Autodesk Fusion 360 part; units mm, degrees
(part 3 of 4)
  spline S239 degree 3 poles (-20.1278, 30.3585) (-20.2422, 30.4762) (-20.3885, 30.5351) (-20.5667, 30.5351) knots 0 0 0 0 1 1 1 1
  line L137 (-20.7879, 29.7232) -> (-20.24, 29.7232)
  spline S240 degree 3 poles (-20.24, 29.7232) (-20.2642, 29.6418) (-20.3043, 29.5768) (-20.3605, 29.5284) knots 0 0 0 0 1 1 1 1
  spline S241 degree 3 poles (-20.3605, 29.5284) (-20.4166, 29.48) (-20.4798, 29.4558) (-20.5502, 29.4558) knots 0 0 0 0 1 1 1 1
  spline S242 degree 3 poles (-20.5502, 29.4558) (-20.6493, 29.4558) (-20.7191, 29.485) (-20.7598, 29.5433) knots 0 0 0 0 1 1 1 1
  spline S243 degree 3 poles (-20.7598, 29.5433) (-20.8005, 29.6016) (-20.8099, 29.6616) (-20.7879, 29.7232) knots 0 0 0 0 1 1 1 1
  line L138 (-22.382, 30.5351) -> (-22.821, 30.4526)
  line L139 (-22.821, 30.4526) -> (-22.821, 30.3833)
  spline S244 degree 3 poles (-22.821, 30.3833) (-22.711, 30.3833) (-22.64, 30.3602) (-22.6081, 30.314) knots 0 0 0 0 1 1 1 1
  spline S245 degree 3 poles (-22.6081, 30.314) (-22.5762, 30.2678) (-22.5603, 30.1621) (-22.5603, 29.9971) knots 0 0 0 0 1 1 1 1
  line L140 (-22.5603, 29.9971) -> (-22.5603, 28.4426)
  line L141 (-22.5603, 28.4426) -> (-22.0652, 28.5251)
  line L142 (-22.0652, 28.5251) -> (-22.0652, 28.5944)
  spline S246 degree 3 poles (-22.0652, 28.5944) (-22.1752, 28.5944) (-22.2462, 28.6175) (-22.2781, 28.6637) knots 0 0 0 0 1 1 1 1
  spline S247 degree 3 poles (-22.2781, 28.6637) (-22.31, 28.7099) (-22.3259, 28.8155) (-22.3259, 28.9806) knots 0 0 0 0 1 1 1 1
  line L143 (-22.3259, 28.9806) -> (-22.3259, 29.5185)
  spline S248 degree 3 poles (-22.3259, 29.5185) (-22.2203, 29.3887) (-22.0861, 29.3238) (-21.9233, 29.3238) knots 0 0 0 0 1 1 1 1
  spline S249 degree 3 poles (-21.9233, 29.3238) (-21.767, 29.3238) (-21.6323, 29.3827) (-21.5189, 29.5004) knots 0 0 0 0 1 1 1 1
  spline S250 degree 3 poles (-21.5189, 29.5004) (-21.4056, 29.6181) (-21.349, 29.7606) (-21.349, 29.9278) knots 0 0 0 0 1 1 1 1
  spline S251 degree 3 poles (-21.349, 29.9278) (-21.349, 30.095) (-21.4056, 30.238) (-21.5189, 30.3569) knots 0 0 0 0 1 1 1 1
  spline S252 degree 3 poles (-21.5189, 30.3569) (-21.6323, 30.4757) (-21.767, 30.5351) (-21.9233, 30.5351) knots 0 0 0 0 1 1 1 1
  spline S253 degree 3 poles (-21.9233, 30.5351) (-22.0861, 30.5351) (-22.2214, 30.468) (-22.3292, 30.3338) knots 0 0 0 0 1 1 1 1
  spline S254 degree 3 poles (-22.3292, 30.3338) (-22.349, 30.435) (-22.3666, 30.5021) (-22.382, 30.5351) knots 0 0 0 0 1 1 1 1
  spline S255 degree 3 poles (-21.9926, 30.4031) (-21.8693, 30.4031) (-21.7758, 30.3591) (-21.712, 30.2711) knots 0 0 0 0 1 1 1 1
  spline S256 degree 3 poles (-21.712, 30.2711) (-21.6482, 30.183) (-21.6163, 30.0686) (-21.6163, 29.9278) knots 0 0 0 0 1 1 1 1
  spline S257 degree 3 poles (-21.6163, 29.9278) (-21.6163, 29.7892) (-21.6482, 29.6759) (-21.712, 29.5878) knots 0 0 0 0 1 1 1 1
  spline S258 degree 3 poles (-21.712, 29.5878) (-21.7758, 29.4998) (-21.8693, 29.4558) (-21.9926, 29.4558) knots 0 0 0 0 1 1 1 1
  spline S259 degree 3 poles (-21.9926, 29.4558) (-22.0652, 29.4558) (-22.1312, 29.4795) (-22.1906, 29.5268) knots 0 0 0 0 1 1 1 1
  spline S260 degree 3 poles (-22.1906, 29.5268) (-22.25, 29.5741) (-22.2951, 29.6374) (-22.3259, 29.7166) knots 0 0 0 0 1 1 1 1
  line L144 (-22.3259, 29.7166) -> (-22.3259, 30.1423)
  spline S261 degree 3 poles (-22.3259, 30.1423) (-22.2951, 30.2215) (-22.25, 30.2848) (-22.1906, 30.3321) knots 0 0 0 0 1 1 1 1
  spline S262 degree 3 poles (-22.1906, 30.3321) (-22.1312, 30.3794) (-22.0652, 30.4031) (-21.9926, 30.4031) knots 0 0 0 0 1 1 1 1
  line L145 (-23.9927, 30.5351) -> (-24.1379, 30.314)
  spline S263 degree 3 poles (-24.1379, 30.314) (-24.2413, 30.4614) (-24.3821, 30.5351) (-24.5604, 30.5351) knots 0 0 0 0 1 1 1 1
  spline S264 degree 3 poles (-24.5604, 30.5351) (-24.7166, 30.5351) (-24.8508, 30.4757) (-24.963, 30.3569) knots 0 0 0 0 1 1 1 1
  spline S265 degree 3 poles (-24.963, 30.3569) (-25.0752, 30.238) (-25.1314, 30.095) (-25.1314, 29.9278) knots 0 0 0 0 1 1 1 1
  spline S266 degree 3 poles (-25.1314, 29.9278) (-25.1314, 29.7606) (-25.0752, 29.6181) (-24.963, 29.5004) knots 0 0 0 0 1 1 1 1
  spline S267 degree 3 poles (-24.963, 29.5004) (-24.8508, 29.3827) (-24.7166, 29.3238) (-24.5604, 29.3238) knots 0 0 0 0 1 1 1 1
  spline S268 degree 3 poles (-24.5604, 29.3238) (-24.3975, 29.3238) (-24.2633, 29.3887) (-24.1577, 29.5185) knots 0 0 0 0 1 1 1 1
  line L146 (-24.1577, 29.5185) -> (-24.1577, 28.4426)
  line L147 (-24.1577, 28.4426) -> (-23.6626, 28.5251)
  line L148 (-23.6626, 28.5251) -> (-23.6626, 28.5944)
  spline S269 degree 3 poles (-23.6626, 28.5944) (-23.7726, 28.5944) (-23.8436, 28.6175) (-23.8755, 28.6637) knots 0 0 0 0 1 1 1 1
  spline S270 degree 3 poles (-23.8755, 28.6637) (-23.9074, 28.7099) (-23.9234, 28.8155) (-23.9234, 28.9806) knots 0 0 0 0 1 1 1 1
  line L149 (-23.9234, 28.9806) -> (-23.9234, 30.5351)
  line L150 (-23.9234, 30.5351) -> (-23.9927, 30.5351)
  spline S271 degree 3 poles (-24.4911, 30.4031) (-24.4162, 30.4031) (-24.3497, 30.3794) (-24.2914, 30.3321) knots 0 0 0 0 1 1 1 1
  spline S272 degree 3 poles (-24.2914, 30.3321) (-24.2331, 30.2848) (-24.1885, 30.2204) (-24.1577, 30.139) knots 0 0 0 0 1 1 1 1
  line L151 (-24.1577, 30.139) -> (-24.1577, 29.7166)
  spline S273 degree 3 poles (-24.1577, 29.7166) (-24.1885, 29.6374) (-24.2331, 29.5741) (-24.2914, 29.5268) knots 0 0 0 0 1 1 1 1
  spline S274 degree 3 poles (-24.2914, 29.5268) (-24.3497, 29.4795) (-24.4162, 29.4558) (-24.4911, 29.4558) knots 0 0 0 0 1 1 1 1
  spline S275 degree 3 poles (-24.4911, 29.4558) (-24.6143, 29.4558) (-24.7078, 29.4998) (-24.7716, 29.5878) knots 0 0 0 0 1 1 1 1
  spline S276 degree 3 poles (-24.7716, 29.5878) (-24.8354, 29.6759) (-24.8673, 29.7892) (-24.8673, 29.9278) knots 0 0 0 0 1 1 1 1
  spline S277 degree 3 poles (-24.8673, 29.9278) (-24.8673, 30.0686) (-24.8354, 30.183) (-24.7716, 30.2711) knots 0 0 0 0 1 1 1 1
  spline S278 degree 3 poles (-24.7716, 30.2711) (-24.7078, 30.3591) (-24.6143, 30.4031) (-24.4911, 30.4031) knots 0 0 0 0 1 1 1 1
  spline S279 degree 3 poles (-25.5637, 31.3701) (-25.6121, 31.3701) (-25.6528, 31.3294) (-25.6858, 31.248) knots 0 0 0 0 1 1 1 1
  line L152 (-25.6858, 31.248) -> (-26.3294, 29.6407)
  spline S280 degree 3 poles (-26.3294, 29.6407) (-26.3822, 29.5108) (-26.4604, 29.4459) (-26.5638, 29.4459) knots 0 0 0 0 1 1 1 1
  line L153 (-26.5638, 29.4459) -> (-26.5638, 29.3799)
  line L154 (-26.5638, 29.3799) -> (-26.1017, 29.3799)
  line L155 (-26.1017, 29.3799) -> (-26.1017, 29.4459)
  spline S281 degree 3 poles (-26.1017, 29.4459) (-26.1699, 29.4459) (-26.2106, 29.4597) (-26.2238, 29.4872) knots 0 0 0 0 1 1 1 1
  spline S282 degree 3 poles (-26.2238, 29.4872) (-26.237, 29.5147) (-26.2282, 29.5658) (-26.1974, 29.6407) knots 0 0 0 0 1 1 1 1
  line L156 (-26.1974, 29.6407) -> (-25.9862, 30.1687)
  line L157 (-25.9862, 30.1687) -> (-25.7452, 29.6407)
  spline S283 degree 3 poles (-25.7452, 29.6407) (-25.71, 29.5592) (-25.7001, 29.5064) (-25.7155, 29.4822) knots 0 0 0 0 1 1 1 1
  spline S284 degree 3 poles (-25.7155, 29.4822) (-25.7309, 29.458) (-25.7761, 29.4459) (-25.8509, 29.4459) knots 0 0 0 0 1 1 1 1
  line L158 (-25.8509, 29.4459) -> (-25.8509, 29.3799)
  line L159 (-25.8509, 29.3799) -> (-25.2667, 29.3799)
  line L160 (-25.2667, 29.3799) -> (-25.2667, 29.4459)
  spline S285 degree 3 poles (-25.2667, 29.4459) (-25.3173, 29.4459) (-25.358, 29.4597) (-25.3888, 29.4872) knots 0 0 0 0 1 1 1 1
  spline S286 degree 3 poles (-25.3888, 29.4872) (-25.4196, 29.5147) (-25.4526, 29.5658) (-25.4878, 29.6407) knots 0 0 0 0 1 1 1 1
  line L161 (-25.4878, 29.6407) -> (-25.8674, 30.4625)
  line L162 (-25.8674, 30.4625) -> (-25.7023, 30.875)
  spline S287 degree 3 poles (-25.7023, 30.875) (-25.6737, 30.9477) (-25.638, 31.0076) (-25.5951, 31.0549) knots 0 0 0 0 1 1 1 1
  spline S288 degree 3 poles (-25.5951, 31.0549) (-25.5522, 31.1022) (-25.5175, 31.1396) (-25.4911, 31.1671) knots 0 0 0 0 1 1 1 1
  spline S289 degree 3 poles (-25.4911, 31.1671) (-25.4647, 31.1946) (-25.4515, 31.226) (-25.4515, 31.2612) knots 0 0 0 0 1 1 1 1
  spline S290 degree 3 poles (-25.4515, 31.2612) (-25.4515, 31.2986) (-25.4631, 31.3261) (-25.4862, 31.3437) knots 0 0 0 0 1 1 1 1
  spline S291 degree 3 poles (-25.4862, 31.3437) (-25.5093, 31.3613) (-25.5351, 31.3701) (-25.5637, 31.3701) knots 0 0 0 0 1 1 1 1
  line L163 (-22, -1.425) -> (-22, 24.075)
  line L164 (-22, 24.075) -> (27.5, 24.075)
  line L165 (27.5, 24.075) -> (27.5, -1.425)
  line L166 (27.5, -1.425) -> (-22, -1.425)
  line L167 (53, -8.5) -> (53, 40.5)
  line L168 (53, 40.5) -> (-53, 40.5)
  line L169 (-53, 40.5) -> (-53, -8.5)
extrude "Extrude7" cut sketch "Sketch10" against normal blind 1 contours L1 L2 L3 S0 S1 L4 L5 L6 S2 S3 L7 L8 L9 L10 L11 S4 S5 S6 S7 | L12 S8 S9 S10 S11 S12 S13 L13 S14 S15 | L16 L17 L18 S19 S20 S21 S22 L19 L20 | L22 L23 L24 S27 S28 S29 S30 L25 L26 | S35 S36 S37 S38 S39 | L27 L28 L29 L30 L31 L32 L33 L34 L35 L36 L37 L38 L39 | L45 S51 S52 S54 S55 L48 | L40 S44 S45 L41 S46 S47 L42 L43 L44 L45 S54 S55 L48 | L42 S48 S49 S50 L43 L45 S51 S52 S53 L46 L47 L48 S56 S57 L49 S58 S59 | L42 S48 S49 S50 L43 L48 | S60 S61 L50 L51 S62 S63 S64 S65 S66 L52 L53 L54 S67 S68 S69 L55 L56 | S70 S71 L57 L58 S72 S73 S74 S75 S76 S77 L59 L60 S78 S79 S80 L61 L62 | S81 S82 L63 L64 S83 S84 S85 L65 L66 S86 S87 S88 L67 L68 | S89 S90 S91 L69 S92 S93 S94 S95 S96 L70 L71 S97 S98 S99 L72 | S100 S101 L73 L74 S102 S103 S104 L75 L76 S105 S106 S107 S108 L77 | S109 S110 S111 L78 S112 S113 S114 S115 S116 L79 L80 S117 S118 S119 L81 | S120 S121 L82 L83 S122 S123 S124 S125 S126 L84 L85 L86 S127 S128 S129 L87 L88 | S130 S131 S132 L89 S133 S134 S135 S136 S137 L90 L91 L92 S138 S139 S140 S141 L93 L94 | S142 S143 S144 L95 S145 S146 S147 L96 L97 S148 S149 S150 S151 L98 L99 bodies 8 in component "GNSS_Enclosure_Top"
hole "Hole4" at (-47.5, 30, 0) at (47.5, 30, 0) at (-47.5, -30, 0) at (47.5, -30, 0) direction (0, 0, -1) diameter 2.1 depth 4 tip angle 180 bodies 7 in component "GNSS_Enclosure_Bottom"
sketch "Sketch8 (2)" plane through (0, 0, 15.7) normal (0, 0, 1) x (-1, 0, 0) in component "GNSS_Enclosure_Bottom"
  line L0 (51, 30) -> (51, -30)
  arc A0 (47.5, -33.5) -> (51, -30) centre (47.5, -30) ccw
  arc A1 (47.5, -33.5) -> (46, -35) centre (47.5, -35) ccw
  arc A2 (42.5, -38.5) -> (46, -35) centre (42.5, -35) ccw
  line L1 (42.5, -38.5) -> (-42.5, -38.5)
  arc A3 (-46, -35) -> (-42.5, -38.5) centre (-42.5, -35) ccw
  arc A4 (-46, -35) -> (-47.5, -33.5) centre (-47.5, -35) ccw
  arc A5 (-51, -30) -> (-47.5, -33.5) centre (-47.5, -30) ccw
  line L2 (-51, -30) -> (-51, 30)
  arc A6 (-47.5, 33.5) -> (-51, 30) centre (-47.5, 30) ccw
  arc A7 (-47.5, 33.5) -> (-46, 35) centre (-47.5, 35) ccw
  arc A8 (-42.5, 38.5) -> (-46, 35) centre (-42.5, 35) ccw
  line L3 (-42.5, 38.5) -> (42.5, 38.5)
  arc A9 (46, 35) -> (42.5, 38.5) centre (42.5, 35) ccw
  arc A10 (46, 35) -> (47.5, 33.5) centre (47.5, 35) ccw
  arc A11 (51, 30) -> (47.5, 33.5) centre (47.5, 30) ccw
  line L4 (-53, -40.5) -> (53, -40.5)
  line L5 (53, -40.5) -> (53, 40.5)
  line L6 (53, 40.5) -> (-53, 40.5)
  line L7 (-53, 40.5) -> (-53, -40.5)
  line L8 (49.5, 37) -> (-49.5, 37)
  line L9 (-49.5, 37) -> (-49.5, -37)
  line L10 (-49.5, -37) -> (49.5, -37)
  line L11 (49.5, -37) -> (49.5, 37)
  point P0 (49.5, -37)
  point P1 (-49.5, -37)
  point P2 (-49.5, 37)
  point P3 (49.5, 37)
  constraint coincident P0 L10.end
  constraint coincident P1 L9.end
  constraint coincident P2 L8.end
  constraint coincident P3 L8.start
hole "Hole5" at (-49.5, 37, 15.7) at (-49.5, -37, 15.7) at (49.5, -37, 15.7) at (49.5, 37, 15.7) direction (0, 0, -1) diameter 2.1 depth 10 tip angle 180 bodies 7 in component "GNSS_Enclosure_Bottom"
fillet "Fillet1'" radius 2 8 edges at (53, -40.5, 5.35) (53, 0, -5) (0, -40.5, -5) (53, 40.5, 5.35) (0, 40.5, -5) (-53, 40.5, 5.35) (-53, 0, -5) (-53, -40.5, 5.35) on bodies 7 in component "GNSS_Enclosure_Bottom"
sketch "Sketch11" plane through (0, 0, 17.7) normal (0, 0, 1) x (-1, 0, 0) in component "GNSS_Enclosure_Top"
  spline S0 degree 3 poles (-34.0203, 31.3378) (-34.6769, 31.3347) (-35.3015, 31.6216) (-35.727, 32.1217) knots 0 0 0 0 1 1 1 1
  line L0 (-35.727, 32.1217) -> (-35.727, 29.2592)
  line L1 (-35.727, 29.2592) -> (-36.3046, 29.2592)
  line L2 (-36.3046, 29.2592) -> (-36.3046, 35.8128)
  line L3 (-36.3046, 35.8128) -> (-35.727, 35.8128)
  line L4 (-35.727, 35.8128) -> (-35.727, 35.099)
  spline S1 degree 3 poles (-35.727, 35.099) (-35.0384, 35.8815) (-33.9048, 36.0931) (-32.9803, 35.6116) knots 0 0 0 0 1 1 1 1
  spline S2 degree 3 poles (-32.9803, 35.6116) (-32.0559, 35.1302) (-31.5794, 34.08) (-31.8258, 33.0672) knots 0 0 0 0 1 1 1 1
  spline S3 degree 3 poles (-31.8258, 33.0672) (-32.0722, 32.0545) (-32.978, 31.3407) (-34.0203, 31.3378) knots 0 0 0 0 1 1 1 1
  spline S4 degree 3 poles (-8.2752, 34.8124) (-8.3121, 34.8143) (-8.3467, 34.8308) (-8.3712, 34.8584) knots -1 -1 -1 -1 0 0 0 0
  line L5 (-8.3712, 34.8584) -> (-9.0609, 35.5522)
  line L6 (-9.0609, 35.5522) -> (-9.0691, 35.5604)
  spline S5 degree 3 poles (-9.0691, 35.5604) (-9.1212, 35.6178) (-9.1175, 35.7063) (-9.0609, 35.7591) knots -1 -1 -1 -1 0 0 0 0
  spline S6 degree 3 poles (-9.0609, 35.7591) (-9.0333, 35.7859) (-8.9962, 35.8005) (-8.9577, 35.7997) knots -1 -1 -1 -1 0 0 0 0
  spline S7 degree 3 poles (-8.9577, 35.7997) (-8.9194, 35.801) (-8.8823, 35.7863) (-8.8553, 35.7591) knots -1 -1 -1 -1 0 0 0 0
  line L7 (-8.8553, 35.7591) -> (-8.2722, 35.1664)
  line L8 (-8.2722, 35.1664) -> (-7.6836, 35.7529)
  line L9 (-7.6836, 35.7529) -> (-7.6726, 35.7646)
  spline S8 degree 3 poles (-7.6726, 35.7646) (-7.6453, 35.789) (-7.6094, 35.8014) (-7.5729, 35.7992) knots -1 -1 -1 -1 0 0 0 0
  spline S9 degree 3 poles (-7.5729, 35.7992) (-7.5363, 35.797) (-7.5022, 35.7804) (-7.478, 35.7529) knots -1 -1 -1 -1 0 0 0 0
  spline S10 degree 3 poles (-7.478, 35.7529) (-7.4745, 35.7501) (-7.4712, 35.7469) (-7.4684, 35.7433) knots -1 -1 -1 -1 0 0 0 0
  spline S11 degree 3 poles (-7.4684, 35.7433) (-7.4429, 35.7161) (-7.4296, 35.6798) (-7.4314, 35.6426) knots -1 -1 -1 -1 0 0 0 0
  spline S12 degree 3 poles (-7.4314, 35.6426) (-7.4332, 35.6054) (-7.45, 35.5705) (-7.478, 35.546) knots -1 -1 -1 -1 0 0 0 0
  line L10 (-7.478, 35.546) -> (-8.1752, 34.8487)
  spline S13 degree 3 poles (-8.1752, 34.8487) (-8.2023, 34.8237) (-8.2384, 34.8106) (-8.2752, 34.8124) knots -1 -1 -1 -1 0 0 0 0
  spline S14 degree 3 poles (-6.3321, 34.0513) (-6.3689, 34.0531) (-6.4035, 34.0696) (-6.428, 34.0972) knots -1 -1 -1 -1 0 0 0 0
  line L11 (-6.428, 34.0972) -> (-7.1225, 34.7855)
  spline S15 degree 3 poles (-7.1225, 34.7855) (-7.1791, 34.8426) (-7.1791, 34.9347) (-7.1225, 34.9918) knots -1 -1 -1 -1 0 0 0 0
  spline S16 degree 3 poles (-7.1225, 34.9918) (-7.1195, 34.9951) (-7.1163, 34.9983) (-7.1129, 35.0014) knots -1 -1 -1 -1 0 0 0 0
  spline S17 degree 3 poles (-7.1129, 35.0014) (-7.0858, 35.0264) (-7.0497, 35.0395) (-7.0129, 35.0377) knots -1 -1 -1 -1 0 0 0 0
  spline S18 degree 3 poles (-7.0129, 35.0377) (-6.976, 35.0359) (-6.9414, 35.0193) (-6.9169, 34.9918) knots -1 -1 -1 -1 0 0 0 0
  line L12 (-6.9169, 34.9918) -> (-6.3283, 34.4045)
  line L13 (-6.3283, 34.4045) -> (-5.7404, 34.9918)
  spline S19 degree 3 poles (-5.7404, 34.9918) (-5.7127, 35.0185) (-5.6757, 35.0333) (-5.6373, 35.033) knots -1 -1 -1 -1 0 0 0 0
  spline S20 degree 3 poles (-5.6373, 35.033) (-5.5789, 35.0342) (-5.5257, 34.9996) (-5.5031, 34.9458) knots -1 -1 -1 -1 0 0 0 0
  spline S21 degree 3 poles (-5.5031, 34.9458) (-5.4805, 34.8919) (-5.493, 34.8297) (-5.5348, 34.7889) knots -1 -1 -1 -1 0 0 0 0
  line L14 (-5.5348, 34.7889) -> (-6.2224, 34.0972)
  line L15 (-6.2224, 34.0972) -> (-6.2321, 34.0875)
  spline S22 degree 3 poles (-6.2321, 34.0875) (-6.2592, 34.0625) (-6.2952, 34.0495) (-6.3321, 34.0513) knots -1 -1 -1 -1 0 0 0 0
  spline S23 degree 3 poles (-4.3851, 33.3478) (-4.4228, 33.349) (-4.4584, 33.3656) (-4.4835, 33.3938) knots -1 -1 -1 -1 0 0 0 0
  line L16 (-4.4835, 33.3938) -> (-5.1745, 34.0862)
  line L17 (-5.1745, 34.0862) -> (-5.1841, 34.0958)
  spline S24 degree 3 poles (-5.1841, 34.0958) (-5.2352, 34.1527) (-5.2315, 34.24) (-5.1759, 34.2925) knots -1 -1 -1 -1 0 0 0 0
  spline S25 degree 3 poles (-5.1759, 34.2925) (-5.1479, 34.3185) (-5.111, 34.333) (-5.0727, 34.333) knots -1 -1 -1 -1 0 0 0 0
  spline S26 degree 3 poles (-5.0727, 34.333) (-5.0344, 34.3344) (-4.9973, 34.3197) (-4.9703, 34.2925) knots -1 -1 -1 -1 0 0 0 0
  line L18 (-4.9703, 34.2925) -> (-4.381, 33.7059)
  line L19 (-4.381, 33.7059) -> (-3.7924, 34.2925)
  spline S27 degree 3 poles (-3.7924, 34.2925) (-3.7652, 34.32) (-3.728, 34.3355) (-3.6893, 34.3355) knots -1 -1 -1 -1 0 0 0 0
  spline S28 degree 3 poles (-3.6893, 34.3355) (-3.6505, 34.3355) (-3.6134, 34.32) (-3.5861, 34.2925) knots -1 -1 -1 -1 0 0 0 0
  spline S29 degree 3 poles (-3.5861, 34.2925) (-3.5295, 34.2354) (-3.5295, 34.1433) (-3.5861, 34.0862) knots -1 -1 -1 -1 0 0 0 0
  line L20 (-3.5861, 34.0862) -> (-4.2779, 33.3938)
  line L21 (-4.2779, 33.3938) -> (-4.2841, 33.3876)
  spline S30 degree 3 poles (-4.2841, 33.3876) (-4.3109, 33.361) (-4.3474, 33.3467) (-4.3851, 33.3478) knots -1 -1 -1 -1 0 0 0 0
  spline S31 degree 3 poles (-4.3851, 34.0512) (-4.4228, 34.0524) (-4.4584, 34.069) (-4.4835, 34.0972) knots -1 -1 -1 -1 0 0 0 0
  line L22 (-4.4835, 34.0972) -> (-5.1848, 34.7985)
  spline S32 degree 3 poles (-5.1848, 34.7985) (-5.2356, 34.8561) (-5.2313, 34.9436) (-5.1752, 34.9959) knots -1 -1 -1 -1 0 0 0 0
  spline S33 degree 3 poles (-5.1752, 34.9959) (-5.1475, 35.0226) (-5.1105, 35.0374) (-5.0721, 35.0371) knots -1 -1 -1 -1 0 0 0 0
  spline S34 degree 3 poles (-5.0721, 35.0371) (-5.0336, 35.0383) (-4.9965, 35.0233) (-4.9696, 34.9959) knots -1 -1 -1 -1 0 0 0 0
  line L23 (-4.9696, 34.9959) -> (-4.3803, 34.4087)
  line L24 (-4.3803, 34.4087) -> (-3.7917, 34.9959)
  spline S35 degree 2 poles (-3.7917, 34.9959) (-3.7883, 35) (-3.7807, 35.0069) knots -1 -1 -1 0 0 0
  spline S36 degree 3 poles (-3.7807, 35.0069) (-3.7535, 35.0313) (-3.7177, 35.0439) (-3.6812, 35.0418) knots -1 -1 -1 -1 0 0 0 0
  spline S37 degree 3 poles (-3.6812, 35.0418) (-3.6446, 35.0397) (-3.6104, 35.0232) (-3.5861, 34.9959) knots -1 -1 -1 -1 0 0 0 0
  spline S38 degree 3 poles (-3.5861, 34.9959) (-3.5828, 34.9928) (-3.5795, 34.9896) (-3.5765, 34.9863) knots -1 -1 -1 -1 0 0 0 0
  spline S39 degree 3 poles (-3.5765, 34.9863) (-3.5511, 34.9591) (-3.5377, 34.9227) (-3.5395, 34.8855) knots -1 -1 -1 -1 0 0 0 0
  spline S40 degree 3 poles (-3.5395, 34.8855) (-3.5413, 34.8483) (-3.5582, 34.8135) (-3.5861, 34.7889) knots -1 -1 -1 -1 0 0 0 0
  line L25 (-3.5861, 34.7889) -> (-4.2841, 34.091)
  spline S41 degree 3 poles (-4.2841, 34.091) (-4.3109, 34.0644) (-4.3474, 34.0501) (-4.3851, 34.0512) knots -1 -1 -1 -1 0 0 0 0
  spline S42 degree 3 poles (-6.3321, 34.8124) (-6.3689, 34.8143) (-6.4035, 34.8308) (-6.428, 34.8584) knots -1 -1 -1 -1 0 0 0 0
  line L26 (-6.428, 34.8584) -> (-7.1232, 35.5467)
  spline S43 degree 3 poles (-7.1232, 35.5467) (-7.1798, 35.6038) (-7.1798, 35.6958) (-7.1232, 35.7529) knots -1 -1 -1 -1 0 0 0 0
  spline S44 degree 3 poles (-7.1232, 35.7529) (-7.0961, 35.7808) (-7.0589, 35.7966) (-7.0201, 35.7966) knots -1 -1 -1 -1 0 0 0 0
  spline S45 degree 3 poles (-7.0201, 35.7966) (-6.9812, 35.7966) (-6.944, 35.7808) (-6.9169, 35.7529) knots -1 -1 -1 -1 0 0 0 0
  line L27 (-6.9169, 35.7529) -> (-6.3283, 35.1664)
  line L28 (-6.3283, 35.1664) -> (-5.7404, 35.7529)
  spline S46 degree 3 poles (-5.7404, 35.7529) (-5.7125, 35.7794) (-5.6757, 35.7944) (-5.6373, 35.7949) knots -1 -1 -1 -1 0 0 0 0
  spline S47 degree 3 poles (-5.6373, 35.7949) (-5.5988, 35.7959) (-5.5616, 35.7807) (-5.5348, 35.7529) knots -1 -1 -1 -1 0 0 0 0
  spline S48 degree 3 poles (-5.5348, 35.7529) (-5.5313, 35.7501) (-5.528, 35.7469) (-5.5252, 35.7433) knots -1 -1 -1 -1 0 0 0 0
  spline S49 degree 3 poles (-5.5252, 35.7433) (-5.4997, 35.7161) (-5.4864, 35.6798) (-5.4882, 35.6426) knots -1 -1 -1 -1 0 0 0 0
  spline S50 degree 3 poles (-5.4882, 35.6426) (-5.49, 35.6054) (-5.5068, 35.5705) (-5.5348, 35.546) knots -1 -1 -1 -1 0 0 0 0
  line L29 (-5.5348, 35.546) -> (-6.2224, 34.8584)
  spline S51 degree 3 poles (-6.2224, 34.8584) (-6.2253, 34.8548) (-6.2285, 34.8516) (-6.2321, 34.8487) knots -1 -1 -1 -1 0 0 0 0
  spline S52 degree 3 poles (-6.2321, 34.8487) (-6.2592, 34.8237) (-6.2952, 34.8106) (-6.3321, 34.8124) knots -1 -1 -1 -1 0 0 0 0
  spline S53 degree 3 poles (-15.2762, 31.3385) (-15.9326, 31.3381) (-16.5356, 31.7006) (-16.8432, 32.2805) knots 0 0 0 0 1 1 1 1
  spline S54 degree 3 poles (-16.8432, 32.2805) (-17.1409, 31.7167) (-17.7371, 31.3385) (-18.4715, 31.3385) knots 0 0 0 0 1 1 1 1
  spline S55 degree 3 poles (-18.4715, 31.3385) (-19.4953, 31.3378) (-20.2661, 32.1657) (-20.2661, 33.2143) knots 0 0 0 0 1 1 1 1
  line L30 (-20.2661, 33.2143) -> (-20.2661, 35.8128)
  line L31 (-20.2661, 35.8128) -> (-19.6706, 35.8128)
  line L32 (-19.6706, 35.8128) -> (-19.6706, 33.2294)
  spline S56 degree 3 poles (-19.6706, 33.2294) (-19.6706, 32.473) (-19.1109, 31.8735) (-18.3752, 31.8735) knots 0 0 0 0 1 1 1 1
  spline S57 degree 3 poles (-18.3752, 31.8735) (-17.6395, 31.8735) (-17.0687, 32.4724) (-17.0687, 33.2294) knots 0 0 0 0 1 1 1 1
  line L33 (-17.0687, 33.2294) -> (-17.0687, 35.8107)
  line L34 (-17.0687, 35.8107) -> (-16.4822, 35.8107)
  line L35 (-16.4822, 35.8107) -> (-16.4822, 33.2294)
  spline S58 degree 3 poles (-16.4822, 33.2294) (-16.4822, 32.473) (-15.9046, 31.8735) (-15.1758, 31.8735) knots 0 0 0 0 1 1 1 1
  spline S59 degree 3 poles (-15.1758, 31.8735) (-14.4469, 31.8735) (-13.8755, 32.473) (-13.8755, 33.2294) knots 0 0 0 0 1 1 1 1
  line L36 (-13.8755, 33.2294) -> (-13.8755, 35.8107)
  line L37 (-13.8755, 35.8107) -> (-13.2979, 35.8107)
  line L38 (-13.2979, 35.8107) -> (-13.2979, 31.4079)
  line L39 (-13.2979, 31.4079) -> (-13.8755, 31.4079)
  line L40 (-13.8755, 31.4079) -> (-13.8755, 32.0605)
  spline S60 degree 3 poles (-13.8755, 32.0605) (-14.2016, 31.6114) (-14.7212, 31.3436) (-15.2762, 31.3385) knots 0 0 0 0 1 1 1 1
  spline S61 degree 3 poles (-41.7621, 33.6287) (-41.7595, 34.8744) (-40.749, 35.8829) (-39.5033, 35.8829) knots 0 0 0 0 1 1 1 1
  spline S62 degree 3 poles (-39.5033, 35.8829) (-38.9019, 35.8827) (-38.3254, 35.6428) (-37.9014, 35.2163) knots 0 0 0 0 1 1 1 1
  spline S63 degree 3 poles (-37.9014, 35.2163) (-37.4775, 34.7897) (-37.241, 34.2117) (-37.2445, 33.6104) knots 0 0 0 0 1 1 1 1
  spline S64 degree 3 poles (-37.2445, 33.6104) (-37.2521, 32.3647) (-38.2667, 31.3603) (-39.5124, 31.3653) knots 0 0 0 0 1 1 1 1
  spline S65 degree 3 poles (-39.5124, 31.3653) (-40.7581, 31.3704) (-41.7646, 32.383) (-41.7621, 33.6287) knots 0 0 0 0 1 1 1 1
  spline S66 degree 3 poles (-28.5814, 31.3378) (-29.238, 31.3347) (-29.8625, 31.6216) (-30.288, 32.1217) knots 0 0 0 0 1 1 1 1
  line L41 (-30.288, 32.1217) -> (-30.288, 31.4079)
  line L42 (-30.288, 31.4079) -> (-30.8656, 31.4079)
  line L43 (-30.8656, 31.4079) -> (-30.8656, 35.8128)
  line L44 (-30.8656, 35.8128) -> (-30.288, 35.8128)
  line L45 (-30.288, 35.8128) -> (-30.288, 35.099)
  spline S67 degree 3 poles (-30.288, 35.099) (-29.5994, 35.8815) (-28.4658, 36.0931) (-27.5413, 35.6116) knots 0 0 0 0 1 1 1 1
  spline S68 degree 3 poles (-27.5413, 35.6116) (-26.6169, 35.1302) (-26.1404, 34.08) (-26.3868, 33.0672) knots 0 0 0 0 1 1 1 1
  spline S69 degree 3 poles (-26.3868, 33.0672) (-26.6333, 32.0545) (-27.5391, 31.3407) (-28.5814, 31.3378) knots 0 0 0 0 1 1 1 1
  spline S70 degree 3 poles (-8.2752, 34.0513) (-8.3121, 34.0531) (-8.3467, 34.0696) (-8.3712, 34.0972) knots -1 -1 -1 -1 0 0 0 0
  line L46 (-8.3712, 34.0972) -> (-9.0609, 34.7889)
  line L47 (-9.0609, 34.7889) -> (-9.0705, 34.7985)
  spline S71 degree 3 poles (-9.0705, 34.7985) (-9.096, 34.8257) (-9.1093, 34.8621) (-9.1075, 34.8992) knots -1 -1 -1 -1 0 0 0 0
  spline S72 degree 3 poles (-9.1075, 34.8992) (-9.1057, 34.9364) (-9.0888, 34.9713) (-9.0609, 34.9959) knots -1 -1 -1 -1 0 0 0 0
  spline S73 degree 3 poles (-9.0609, 34.9959) (-9.0334, 35.0228) (-8.9962, 35.0377) (-8.9577, 35.0371) knots -1 -1 -1 -1 0 0 0 0
  spline S74 degree 3 poles (-8.9577, 35.0371) (-8.9193, 35.0383) (-8.8822, 35.0233) (-8.8553, 34.9959) knots -1 -1 -1 -1 0 0 0 0
  line L48 (-8.8553, 34.9959) -> (-8.2722, 34.4087)
  line L49 (-8.2722, 34.4087) -> (-7.6836, 34.9959)
  line L50 (-7.6836, 34.9959) -> (-7.6802, 34.9959)
  spline S75 degree 3 poles (-7.6802, 34.9959) (-7.6534, 35.0228) (-7.617, 35.038) (-7.5791, 35.038) knots -1 -1 -1 -1 0 0 0 0
  spline S76 degree 3 poles (-7.5791, 35.038) (-7.5411, 35.038) (-7.5047, 35.0228) (-7.478, 34.9959) knots -1 -1 -1 -1 0 0 0 0
  spline S77 degree 3 poles (-7.478, 34.9959) (-7.4746, 34.9928) (-7.4714, 34.9896) (-7.4684, 34.9863) knots -1 -1 -1 -1 0 0 0 0
  spline S78 degree 3 poles (-7.4684, 34.9863) (-7.4429, 34.9591) (-7.4296, 34.9227) (-7.4314, 34.8855) knots -1 -1 -1 -1 0 0 0 0
  spline S79 degree 3 poles (-7.4314, 34.8855) (-7.4332, 34.8483) (-7.45, 34.8135) (-7.478, 34.7889) knots -1 -1 -1 -1 0 0 0 0
  line L51 (-7.478, 34.7889) -> (-8.1656, 34.0972)
  spline S80 degree 3 poles (-8.1656, 34.0972) (-8.1691, 34.0943) (-8.1724, 34.0911) (-8.1752, 34.0875) knots -1 -1 -1 -1 0 0 0 0
  spline S81 degree 3 poles (-8.1752, 34.0875) (-8.2023, 34.0625) (-8.2384, 34.0495) (-8.2752, 34.0513) knots -1 -1 -1 -1 0 0 0 0
  spline S82 degree 3 poles (-6.3321, 33.3478) (-6.3689, 33.3497) (-6.4035, 33.3662) (-6.428, 33.3938) knots -1 -1 -1 -1 0 0 0 0
  line L52 (-6.428, 33.3938) -> (-7.1094, 34.0869)
  spline S83 degree 3 poles (-7.1094, 34.0869) (-7.1653, 34.1443) (-7.1653, 34.2357) (-7.1094, 34.2931) knots -1 -1 -1 -1 0 0 0 0
  spline S84 degree 3 poles (-7.1094, 34.2931) (-7.0822, 34.3207) (-7.045, 34.3362) (-7.0063, 34.3362) knots -1 -1 -1 -1 0 0 0 0
  spline S85 degree 3 poles (-7.0063, 34.3362) (-6.9675, 34.3362) (-6.9304, 34.3207) (-6.9032, 34.2931) knots -1 -1 -1 -1 0 0 0 0
  line L53 (-6.9032, 34.2931) -> (-6.3166, 33.7066)
  line L54 (-6.3166, 33.7066) -> (-5.7404, 34.2931)
  spline S86 degree 3 poles (-5.7404, 34.2931) (-5.7124, 34.3192) (-5.6755, 34.3337) (-5.6373, 34.3337) knots -1 -1 -1 -1 0 0 0 0
  spline S87 degree 3 poles (-5.6373, 34.3337) (-5.5991, 34.3344) (-5.5622, 34.3198) (-5.5348, 34.2931) knots -1 -1 -1 -1 0 0 0 0
  spline S88 degree 3 poles (-5.5348, 34.2931) (-5.5314, 34.2901) (-5.5282, 34.2869) (-5.5252, 34.2835) knots -1 -1 -1 -1 0 0 0 0
  spline S89 degree 3 poles (-5.5252, 34.2835) (-5.4997, 34.2563) (-5.4864, 34.22) (-5.4882, 34.1828) knots -1 -1 -1 -1 0 0 0 0
  spline S90 degree 3 poles (-5.4882, 34.1828) (-5.49, 34.1456) (-5.5068, 34.1107) (-5.5348, 34.0862) knots -1 -1 -1 -1 0 0 0 0
  line L55 (-5.5348, 34.0862) -> (-6.2224, 33.3938)
  spline S91 degree 3 poles (-6.2224, 33.3938) (-6.2255, 33.3904) (-6.2287, 33.3872) (-6.2321, 33.3841) knots -1 -1 -1 -1 0 0 0 0
  spline S92 degree 3 poles (-6.2321, 33.3841) (-6.2592, 33.3591) (-6.2952, 33.346) (-6.3321, 33.3478) knots -1 -1 -1 -1 0 0 0 0
  line L56 (-6.5614, 28.5028) -> (-11.5892, 35.3321)
  spline S93 degree 3 poles (-11.5892, 35.3321) (-11.6866, 35.4643) (-11.6593, 35.6502) (-11.528, 35.7488) knots 0 0 0 0 1 1 1 1
  spline S94 degree 3 poles (-11.528, 35.7488) (-11.4774, 35.7867) (-11.4159, 35.8072) (-11.3527, 35.8073) knots 0 0 0 0 1 1 1 1
  spline S95 degree 3 poles (-11.3527, 35.8073) (-11.2587, 35.8073) (-11.1704, 35.7626) (-11.1148, 35.6869) knots 0 0 0 0 1 1 1 1
  line L57 (-11.1148, 35.6869) -> (-6.3242, 29.1794)
  line L58 (-6.3242, 29.1794) -> (-1.5492, 35.6657)
  spline S96 degree 3 poles (-1.5492, 35.6657) (-1.4968, 35.7507) (-1.4029, 35.8073) (-1.2957, 35.8073) knots 0.348422 0.348422 0.348422 0.348422 1 1 1 1
  line L59 (-1.2957, 35.8073) -> (3.6551, 35.8073)
  spline S97 degree 3 poles (3.6551, 35.8073) (3.767, 35.8073) (3.8693, 35.7438) (3.9191, 35.6436) knots 0 0 0 0 1 1 1 1
  spline S98 degree 3 poles (3.9191, 35.6436) (3.969, 35.5429) (3.9586, 35.4228) (3.8923, 35.3321) knots 0 0 0 0 1 1 1 1
  line L60 (3.8923, 35.3321) -> (-1.1369, 28.5028)
  spline S99 degree 3 poles (-1.1369, 28.5028) (-1.1924, 28.4273) (-1.2804, 28.3826) (-1.3741, 28.3825) knots 0 0 0 0 1 1 1 1
  spline S100 degree 3 poles (-1.3741, 28.3825) (-1.4668, 28.3835) (-1.5537, 28.4281) (-1.6086, 28.5028) knots 0 0 0 0 1 1 1 1
  line L61 (-1.6086, 28.5028) -> (-3.8481, 31.5443)
  line L62 (-3.8481, 31.5443) -> (-6.087, 28.5028)
  spline S101 degree 3 poles (-6.087, 28.5028) (-6.1424, 28.4273) (-6.2305, 28.3827) (-6.3242, 28.3827) knots 0 0 0 0 1 1 1 1
  spline S102 degree 3 poles (-6.3242, 28.3827) (-6.4179, 28.3827) (-6.506, 28.4273) (-6.5614, 28.5028) knots 0 0 0 0 1 1 1 1
  spline S103 degree 3 poles (-4.3852, 34.8121) (-4.4229, 34.8134) (-4.4585, 34.8301) (-4.4835, 34.8584) knots -1 -1 -1 -1 0 0 0 0
  line L63 (-4.4835, 34.8584) -> (-5.1752, 35.546)
  line L64 (-5.1752, 35.546) -> (-5.1848, 35.5556)
  spline S104 degree 3 poles (-5.1848, 35.5556) (-5.236, 35.613) (-5.2317, 35.7008) (-5.1752, 35.7529) knots -1 -1 -1 -1 0 0 0 0
  spline S105 degree 3 poles (-5.1752, 35.7529) (-5.1473, 35.7794) (-5.1105, 35.7944) (-5.0721, 35.7949) knots -1 -1 -1 -1 0 0 0 0
  spline S106 degree 3 poles (-5.0721, 35.7949) (-5.0335, 35.7959) (-4.9964, 35.7807) (-4.9696, 35.7529) knots -1 -1 -1 -1 0 0 0 0
  line L65 (-4.9696, 35.7529) -> (-4.3803, 35.1664)
  line L66 (-4.3803, 35.1664) -> (-3.7917, 35.7529)
  line L67 (-3.7917, 35.7529) -> (-3.7807, 35.7646)
  spline S107 degree 3 poles (-3.7807, 35.7646) (-3.7534, 35.789) (-3.7175, 35.8014) (-3.681, 35.7992) knots -1 -1 -1 -1 0 0 0 0
  spline S108 degree 3 poles (-3.681, 35.7992) (-3.6445, 35.797) (-3.6103, 35.7804) (-3.5861, 35.7529) knots -1 -1 -1 -1 0 0 0 0
  spline S109 degree 3 poles (-3.5861, 35.7529) (-3.5826, 35.7501) (-3.5794, 35.7469) (-3.5765, 35.7433) knots -1 -1 -1 -1 0 0 0 0
  spline S110 degree 3 poles (-3.5765, 35.7433) (-3.5511, 35.7161) (-3.5377, 35.6798) (-3.5395, 35.6426) knots -1 -1 -1 -1 0 0 0 0
  spline S111 degree 3 poles (-3.5395, 35.6426) (-3.5413, 35.6054) (-3.5582, 35.5705) (-3.5861, 35.546) knots -1 -1 -1 -1 0 0 0 0
  line L68 (-3.5861, 35.546) -> (-4.2779, 34.8584)
  line L69 (-4.2779, 34.8584) -> (-4.2841, 34.8515)
  spline S112 degree 3 poles (-4.2841, 34.8515) (-4.311, 34.825) (-4.3475, 34.8108) (-4.3852, 34.8121) knots -1 -1 -1 -1 0 0 0 0
  spline S113 degree 3 poles (-8.2752, 33.3478) (-8.3121, 33.3497) (-8.3467, 33.3662) (-8.3712, 33.3938) knots -1 -1 -1 -1 0 0 0 0
  line L70 (-8.3712, 33.3938) -> (-9.0616, 34.0855)
  line L71 (-9.0616, 34.0855) -> (-9.0712, 34.0951)
  spline S114 degree 3 poles (-9.0712, 34.0951) (-9.0966, 34.1223) (-9.11, 34.1586) (-9.1082, 34.1958) knots -1 -1 -1 -1 0 0 0 0
  spline S115 degree 3 poles (-9.1082, 34.1958) (-9.1064, 34.233) (-9.0895, 34.2679) (-9.0616, 34.2925) knots -1 -1 -1 -1 0 0 0 0
  spline S116 degree 3 poles (-9.0616, 34.2925) (-9.0336, 34.3187) (-8.9967, 34.3332) (-8.9584, 34.333) knots -1 -1 -1 -1 0 0 0 0
  spline S117 degree 3 poles (-8.9584, 34.333) (-8.9201, 34.3344) (-8.883, 34.3197) (-8.856, 34.2925) knots -1 -1 -1 -1 0 0 0 0
  line L72 (-8.856, 34.2925) -> (-8.2729, 33.7059)
  line L73 (-8.2729, 33.7059) -> (-7.6843, 34.2925)
  spline S118 degree 3 poles (-7.6843, 34.2925) (-7.657, 34.32) (-7.6199, 34.3355) (-7.5811, 34.3355) knots -1 -1 -1 -1 0 0 0 0
  spline S119 degree 3 poles (-7.5811, 34.3355) (-7.5424, 34.3355) (-7.5052, 34.32) (-7.478, 34.2925) knots -1 -1 -1 -1 0 0 0 0
  spline S120 degree 3 poles (-7.478, 34.2925) (-7.4214, 34.2354) (-7.4214, 34.1433) (-7.478, 34.0862) knots -1 -1 -1 -1 0 0 0 0
  line L74 (-7.478, 34.0862) -> (-8.1656, 33.3938)
  spline S121 degree 3 poles (-8.1656, 33.3938) (-8.169, 33.3907) (-8.1722, 33.3875) (-8.1752, 33.3841) knots -1 -1 -1 -1 0 0 0 0
  spline S122 degree 3 poles (-8.1752, 33.3841) (-8.2023, 33.3591) (-8.2384, 33.346) (-8.2752, 33.3478) knots -1 -1 -1 -1 0 0 0 0
  line L75 (-25.593, 33.4054) -> (-21.7679, 34.1041)
  spline S123 degree 3 poles (-21.7679, 34.1041) (-21.9694, 34.811) (-22.6142, 35.2994) (-23.3493, 35.3019) knots 0 0 0 0 1 1 1 1
  spline S124 degree 3 poles (-23.3493, 35.3019) (-24.1745, 35.3019) (-24.8318, 34.738) (-25.0333, 34.1831) knots 0 0 0 0 1 1 1 1
  line L76 (-25.0333, 34.1831) -> (-25.5229, 34.3592)
  spline S125 degree 3 poles (-25.5229, 34.3592) (-25.2953, 34.978) (-24.5341, 35.8478) (-23.3521, 35.8396) knots 0 0 0 0 1 1 1 1
  spline S126 degree 3 poles (-23.3521, 35.8396) (-22.3516, 35.8248) (-21.4748, 35.1666) (-21.1813, 34.2099) knots 0 0 0 0 1 1 1 1
  spline S127 degree 3 poles (-21.1813, 34.2099) (-21.121, 34.0032) (-21.0913, 33.7886) (-21.0933, 33.5732) knots 0 0 0 0 1 1 1 1
  spline S128 degree 3 poles (-21.0933, 33.5732) (-21.0779, 32.3729) (-22.0065, 31.3713) (-23.2046, 31.2961) knots 0 0 0 0 1 1 1 1
  spline S129 degree 3 poles (-23.2046, 31.2961) (-24.4027, 31.2209) (-25.4492, 32.0985) (-25.5841, 33.2913) knots 0 0 0 0 1 1 1 1
  spline S130 degree 3 poles (-25.5841, 33.2913) (-25.5912, 33.3289) (-25.5942, 33.3672) (-25.593, 33.4054) knots 0 0 0 0 1 1 1 1
  line L77 (-45.6684, 31.4079) -> (-46.9295, 34.9938)
  line L78 (-46.9295, 34.9938) -> (-48.1898, 31.4079)
  line L79 (-48.1898, 31.4079) -> (-48.7784, 31.4079)
  line L80 (-48.7784, 31.4079) -> (-47.2293, 35.8128)
  line L81 (-47.2293, 35.8128) -> (-46.6469, 35.8128)
  line L82 (-46.6469, 35.8128) -> (-45.4092, 32.1836)
  line L83 (-45.4092, 32.1836) -> (-44.1715, 35.8128)
  line L84 (-44.1715, 35.8128) -> (-43.5939, 35.8128)
  line L85 (-43.5939, 35.8128) -> (-42.0536, 31.4079)
  line L86 (-42.0536, 31.4079) -> (-42.6312, 31.4079)
  line L87 (-42.6312, 31.4079) -> (-43.8834, 34.9938)
  line L88 (-43.8834, 34.9938) -> (-45.1437, 31.4079)
  line L89 (-45.1437, 31.4079) -> (-45.6684, 31.4079)
  line L90 (-53, -8.5) -> (53, -8.5)
  line L91 (53, -8.5) -> (53, 40.5)
  line L92 (53, 40.5) -> (-53, 40.5)
  line L93 (-53, 40.5) -> (-53, -8.5)
  line L94 (-22, -1.425) -> (-22, 24.075)
  line L95 (-22, 24.075) -> (27.5, 24.075)
  line L96 (27.5, 24.075) -> (27.5, -1.425)
  line L97 (27.5, -1.425) -> (-22, -1.425)
  point P0 (49.5, 37)
  point P1 (-49.5, 37)
hole "Hole3" at (-49.5, -37, 17.7) at (49.5, -37, 17.7) direction (0, 0, -1) diameter 2.1 end up to surface (2 mm away) counterbore diameter 3.6 counterbore depth 1 bodies 8 in component "GNSS_Enclosure_Top"
sketch "Sketch12" plane through (0, 0, 24.2) normal (0, 0, 1) x (-1, 0, 0) in component "GNSS_Enclosure_Top"
  line L0 (53, -8.5) -> (-53, -8.5)
  line L1 (-53, -8.5) -> (-53, -40.5)
  line L2 (-53, -40.5) -> (53, -40.5)
  line L3 (53, -40.5) -> (53, -8.5)
  point P0 (49.5, -37)
  point P1 (-49.5, -37)
hole "Hole4'" at (-49.5, 37, 24.2) at (49.5, 37, 24.2) direction (0, 0, -1) diameter 2.1 end up to surface (8.5 mm away) counterbore diameter 3.6 counterbore depth 2 bodies 8 in component "GNSS_Enclosure_Top"
fillet "Fillet4" radius 2 4 edges at (53, -40.5, 16.7) (53, 40.5, 19.95) (-53, 40.5, 19.95) (-53, -40.5, 16.7) on bodies 8 in component "GNSS_Enclosure_Top"
fillet "Fillet5" radius 1.9 13 edges at (-53, -15, 17.7) (-52.4142, -39.9142, 17.7) (0, -40.5, 17.7) (52.4142, -39.9142, 17.7) (53, -15, 17.7) (0, 8.5, 24.2) (-53, 8.5, 20.95) (53, 8.5, 20.95) (53, 23.5, 24.2) (52.4142, 39.9142, 24.2) (0, 40.5, 24.2) (-52.4142, 39.9142, 24.2) (-53, 23.5, 24.2) on bodies 8 in component "GNSS_Enclosure_Top"
chamfer "Chamfer4" distance 1.5 angle 45 4 edges at (-27.5, -11.325, 17.7) (-2.75, 1.425, 17.7) (22, -11.325, 17.7) (-2.75, -24.075, 17.7) on bodies 8 in component "GNSS_Enclosure_Top"
component "GNSS_PCB" placed x (1, 0, 0) y (0, 1, 0) z (0, 0, 1) at (0, 0, 0)
component "GNSS_Enclosure_Bottom" placed x (1, 0, 0) y (0, 1, 0) z (0, 0, 1) at (0, 0, 0)
component "GNSS_Enclosure_Top" placed x (1, 0, 0) y (0, 1, 0) z (0, 0, 1) at (0, 0, 0)
hidden bodies 2 4 5 6
equation "PCB_X_Size = 100 mm"
equation "PCB_Y_Size = 75 mm"
equation "PCB_Bolt_Inset = 2.5 mm"
equation "PCB_Z_Size = 1.7 mm"
equation "d6 = PCB_Y_Size + ( PCB_Y_Size * PCB_Shrinkage_Percent )"
equation "PCB_Shrinkage_Percent = 0.000"
equation "d8 = PCB_X_Size + ( PCB_X_Size * PCB_Shrinkage_Percent )"
equation "Screen_PCB_X_Size = 61 mm"
equation "Screen_PCB_Y_Size = 39.5 mm"
equation "Screen_DisplayArea_X_Size = 49.5 mm"
equation "Screen_DisplayArea_Y_Size = 25.5 mm"
equation "Screen_DisplayArea_X_Offset = 3 mm"
equation "Screen_DisplayArea_Y_Offset = 7.5 mm"
equation "Screen_Center_X_Offset = 0 mm"
equation "Screen_Center_Y_Offset = -11.325 mm"
equation "d19 = Screen_PCB_X_Size"
equation "d20 = Screen_PCB_Y_Size"
equation "d21 = ( Screen_PCB_X_Size / 2 ) + Screen_Center_X_Offset"
equation "d22 = ( Screen_PCB_Y_Size / 2 ) + Screen_Center_Y_Offset"
equation "d23 = Screen_DisplayArea_X_Size"
equation "d24 = Screen_DisplayArea_Y_Size"
equation "d25 = ( Screen_PCB_Y_Size - Screen_DisplayArea_Y_Size ) / 2"
equation "d26 = Screen_DisplayArea_X_Offset"
equation "BatteryHolder_X_Size = 77 mm"
equation "BatteryHolder_Y_Size = 20.65 mm"
equation "BatteryHolder_Z_Size = 18.5 mm"
equation "d30 = BatteryHolder_X_Size"
equation "d31 = BatteryHolder_Y_Size"
equation "d32 = ( BatteryHolder_X_Size / 2 ) + BatteryHolder_Center_X_Offset"
equation "BatteryHolder_Center_X_Offset = 0 mm"
equation "BatteryHolder_Center_Y_Offset = 25.5 mm"
equation "d35 = ( BatteryHolder_Y_Size / 2 ) + BatteryHolder_Center_Y_Offset"
equation "USB_X_Center_Offset = 17 mm"
equation "SolarInput_X_CenterOffset = 12 mm"
equation "d38 = USB_X_Center_Offset"
equation "d39 = SolarInput_X_CenterOffset"
equation "USB_Jack_X_Size = 9 mm"
equation "USB_Jack_Z_Size = 3.4 mm"
equation "USB_Jack_Y_Size = 7.4 mm"
equation "d43 = USB_Jack_X_Size"
equation "d44 = USB_Jack_Y_Size"
equation "d45 = USB_Jack_Y_Size"
equation "SolarInput_X_Size = 5.5 mm"
equation "SolarInput_Y_Size = 12 mm"
equation "SolarInput_Z_Size = 7.5 mm"
equation "d49 = SolarInput_X_Size"
equation "d50 = SolarInput_Y_Size"
equation "d51 = SolarInput_Y_Size - SolarInput_EdgeOverhang"
equation "SolarInput_EdgeOverhang = 3 mm"